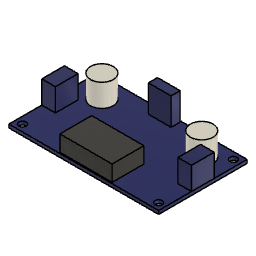
DC模块 v2 (Autodesk Fusion 360 design; units mm, degrees)
Autodesk Fusion 360 part; units mm, degrees
sketch "草图1" plane through (0, 0, 0) normal (0, 0, 1) x (1, 0, 0)
  line L0 (0, 0) -> (66, 0)
  line L1 (66, 0) -> (66, 39)
  line L2 (66, 39) -> (0, 39)
  line L3 (0, 39) -> (0, 0)
  line L4 (-18.8664, 19.5) -> (92.9344, 19.5)
  line L5 (33, 51.4326) -> (33, -27.2938)
  circle A0 centre (3, 36) radius 1.6
  circle A1 centre (63, 36) radius 1.6
  circle A2 centre (3, 3) radius 1.6
  circle A3 centre (63, 3) radius 1.6
  dimension "d1" = 66
  dimension "d2" = 39
  dimension "d3" = 3.2
  dimension "d4" = 60
  dimension "d5" = 33
  constraint horizontal L0
  constraint vertical L1
  constraint horizontal L2
  constraint vertical L3
  constraint coincident L0.start L3.end
  constraint horizontal L4
  constraint perpendicular L4 L5
  constraint symmetric L0 L2 L4
  constraint symmetric L5 A0 A1
  constraint symmetric L4 A0 A2
  constraint symmetric L4 A1 A3
  measures "d1" distance of L0.start L0.end
  measures "d2" distance of L0.start L2.end
  measures "d3" diameter of A0
  measures "d4" distance of A2.centre A3.centre
  measures "d5" distance of A0.centre A2.centre
extrude "拉伸1" add sketch "草图1" along normal blind 1.5 makes body 1
sketch "草图2" plane through (0, 0, 1.5) normal (0, 0, 1) x (-1, 0, 0)
  circle A0 centre (-3, -36) radius 1.6
  circle A1 centre (-63, -3) radius 1.6
  circle A2 centre (-3, -3) radius 1.6
  circle A3 centre (-63, -36) radius 1.6
  line L0 (0, -39) -> (0, 0)
  line L1 (0, 0) -> (-66, 0)
  line L2 (-66, 0) -> (-66, -39)
  line L3 (-66, -39) -> (0, -39)
  line L4 (0, -24.5) -> (-6, -24.5)
  line L5 (-6, -24.5) -> (-6, -14.5)
  line L6 (-6, -14.5) -> (0, -14.5)
  line L7 (0, -14.5) -> (0, -24.5)
  line L8 (-66, -24.5) -> (-60, -24.5)
  line L9 (-60, -24.5) -> (-60, -14.5)
  line L10 (-60, -14.5) -> (-66, -14.5)
  line L11 (-66, -14.5) -> (-66, -24.5)
  dimension "d8" = 10
  dimension "d9" = 10
  dimension "d10" = 6
  dimension "d11" = 6
  dimension "d12" = 14.5
  dimension "d13" = 14.5
  constraint horizontal L4
  constraint vertical L5
  constraint horizontal L6
  constraint vertical L7
  constraint coincident L0 L4.start
  constraint horizontal L8
  constraint vertical L9
  constraint horizontal L10
  constraint vertical L11
  constraint coincident L2 L8.start
  measures "d8" distance of L4.end L5.end
  measures "d9" distance of L8.end L9.end
  measures "d10" distance of L4.start L4.end
  measures "d11" distance of L8.start L8.end
  measures "d12" distance of L3 L4
  measures "d13" distance of L3 L8
extrude "拉伸2" add sketch "草图2" along normal blind 10 separate body contours L0 L4 L5 L6 L7 | L2 L8 L9 L10 L11 makes body 2 at (6, 21.1667, 4.8333) makes body 3 at (66, 17.8333, 4.8333)
sketch "草图3" plane through (0, 0, 1.5) normal (0, 0, 1) x (-1, 0, 0)
  circle A0 centre (-3, -36) radius 1.6
  circle A1 centre (-63, -3) radius 1.6
  circle A2 centre (-3, -3) radius 1.6
  circle A3 centre (-63, -36) radius 1.6
  line L0 (0, -39) -> (0, 0)
  line L1 (0, 0) -> (-66, 0)
  line L2 (-66, 0) -> (-66, -39)
  line L3 (-66, -39) -> (0, -39)
  circle A4 centre (-11, -30) radius 5
  circle A5 centre (-55, -30) radius 5
  dimension "d16" = 10
  dimension "d17" = 10
  dimension "d18" = 11
  dimension "d19" = 11
  dimension "d20" = 9
  dimension "d21" = 9
  measures "d16" diameter of A4
  measures "d17" diameter of A5
  measures "d18" distance of L0 A4.centre
  measures "d19" distance of L2 A5.centre
  measures "d20" distance of L3 A4.centre
  measures "d21" distance of L3 A5.centre
extrude "拉伸3" add sketch "草图3" along normal blind 10 separate body contours A4 | A5 makes body 4 at (50.0062, 30.2492, 8.1667) makes body 5 at (6.0062, 30.2492, 8.1667)
sketch "草图4" plane through (0, 0, 1.5) normal (0, 0, 1) x (-1, 0, 0)
  circle A0 centre (-3, -36) radius 1.6
  circle A1 centre (-63, -3) radius 1.6
  circle A2 centre (-3, -3) radius 1.6
  circle A3 centre (-63, -36) radius 1.6
  line L0 (0, -39) -> (0, 0)
  line L1 (0, 0) -> (-66, 0)
  line L2 (-66, 0) -> (-66, -39)
  line L3 (-66, -39) -> (0, -39)
  line L4 (-27, -38.5) -> (-37, -38.5)
  line L5 (-37, -38.5) -> (-37, -34.5)
  line L6 (-37, -34.5) -> (-27, -34.5)
  line L7 (-27, -34.5) -> (-27, -38.5)
  dimension "d24" = 10
  dimension "d25" = 4
  dimension "d26" = 27
  dimension "d27" = 0.5
  constraint horizontal L4
  constraint vertical L5
  constraint horizontal L6
  constraint vertical L7
  measures "d24" distance of L5.end L6.end
  measures "d25" distance of L4.end L5.end
  measures "d26" distance of L0 L7
  measures "d27" distance of L3 L4
extrude "拉伸4" add sketch "草图4" along normal blind 12 separate body contours L4 L5 L6 L7 makes body 6
sketch "草图5" plane through (0, 0, 1.5) normal (0, 0, 1) x (-1, 0, 0)
  circle A0 centre (-3, -36) radius 1.6
  circle A1 centre (-63, -3) radius 1.6
  circle A2 centre (-3, -3) radius 1.6
  circle A3 centre (-63, -36) radius 1.6
  line L0 (0, -39) -> (0, 0)
  line L1 (0, 0) -> (-66, 0)
  line L2 (-66, 0) -> (-66, -39)
  line L3 (-66, -39) -> (0, -39)
  line L4 (-22, -14.5) -> (-45, -14.5)
  line L5 (-45, -14.5) -> (-45, -0.5)
  line L6 (-45, -0.5) -> (-22, -0.5)
  line L7 (-22, -0.5) -> (-22, -14.5)
  dimension "d30" = 23
  dimension "d31" = 14
  dimension "d32" = 21
  dimension "d33" = 0.5
  constraint horizontal L4
  constraint vertical L5
  constraint horizontal L6
  constraint vertical L7
  measures "d30" distance of L4.start L4.end
  measures "d31" distance of L4.start L6.end
  measures "d32" distance of L2 L5
  measures "d33" distance of L1 L6
extrude "拉伸5" add sketch "草图5" along normal blind 7 separate body contours L4 L5 L6 L7 makes body 7
copy_body "实体->零部件1" bodies 1 removing the originals makes body 8 in component "Component'"
copy_body "实体->零部件2" bodies 2 removing the originals makes body 9 in component "Component''"
copy_body "实体->零部件3" bodies 3 removing the originals makes body 10 in component "Component'''"
copy_body "实体->零部件4" bodies 4 removing the originals makes body 11 in component "Component''''"
copy_body "实体->零部件5" bodies 5 removing the originals makes body 12 in component "Component'''''"
copy_body "实体->零部件6" bodies 6 removing the originals makes body 13 in component "Component''''''"
copy_body "实体->零部件7" bodies 7 removing the originals makes body 14 in component "Component'''''''"
component "Component'" placed x (1, 0, 0) y (0, 1, 0) z (0, 0, 1) at (0, 0, 0)
component "Component''" placed x (1, 0, 0) y (0, 1, 0) z (0, 0, 1) at (0, 0, 0)
component "Component'''" placed x (1, 0, 0) y (0, 1, 0) z (0, 0, 1) at (0, 0, 0)
component "Component''''" placed x (1, 0, 0) y (0, 1, 0) z (0, 0, 1) at (0, 0, 0)
component "Component'''''" placed x (1, 0, 0) y (0, 1, 0) z (0, 0, 1) at (0, 0, 0)
component "Component''''''" placed x (1, 0, 0) y (0, 1, 0) z (0, 0, 1) at (0, 0, 0)
component "Component'''''''" placed x (1, 0, 0) y (0, 1, 0) z (0, 0, 1) at (0, 0, 0)
